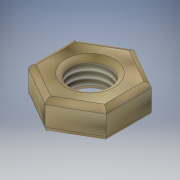
# Autodesk Inventor part: Nut
Saved by Autodesk Inventor 2019 (Build 230136000, 136)
## iProperties
Created: 2019-03-17
Part Number: Nut
Material: Generic
Document SubType Name: Modeling
Designer: Jared
Density: 1 g/cm^3
Appearance: Plaid - Beige
Author: Jared
Autodesk Inventor part; units mm, degrees
ref_plane "YZ Plane" through (0, 0, 0) normal (1, 0, 0) x (0, 1, 0)
ref_plane "XZ Plane" through (0, 0, 0) normal (0, 1, 0) x (-1, 0, 0)
ref_plane "XY Plane" through (0, 0, 0) normal (0, 0, 1) x (1, 0, 0)
sketch "Sketch1" plane through (0, 0, 0) normal (0, 1, 0) x (-1, 0, 0)
  line L0 (4, -2.3094) -> (0, -4.6188)
  line L1 (0, -4.6188) -> (-4, -2.3094)
  line L2 (-4, -2.3094) -> (-4, 2.3094)
  line L3 (-4, 2.3094) -> (0, 4.6188)
  line L4 (0, 4.6188) -> (4, 2.3094)
  line L5 (4, 2.3094) -> (4, -2.3094)
  circle A0 centre (0, 0) radius 2
  dimension "d0" = 4
  dimension "d4" = 4
  constraints: 12 end point, 2 coincident, 1 centre point, 13 other
  measures "d0" distance from line of L5 point (0, 0)
  measures "d4" diameter of A0
extrude "Extrusion1" add sketch "Sketch1" along normal blind 3
fillet "Fillet1" radius 0.5 14 edges at (4, 3, 0) (2, 3, -3.4641) (-2, 3, -3.4641) (-4, 3, 0) (-2, 3, 3.4641) (2, 3, 3.4641) (2, 0, 3.4641) (-2, 0, 3.4641) (4, 0, 0) (-4, 0, 0) (-2, 0, -3.4641) (2, 0, -3.4641) (2, 3, 0) (2, 0, 0)
thread "Thread1" size "M4x0.7" class "6H" standard "ANSI Metric M Profile" full length
body "Solid1"
